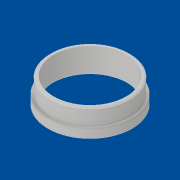
# Autodesk Inventor part: 106-pulley adapter
Saved by Autodesk Inventor 2018 (Build 220112000, 112)
## iProperties
Created: 2020-09-07
Part Number: 106-pulley adapter
Material: Generic
Document SubType Name: Modeling
Designer: Bunny320
Density: 1 g/cm^3
Appearance: Default
Author: Bunny320
Autodesk Inventor part; units mm, degrees
ref_plane "YZ Plane" through (0, 0, 0) normal (1, 0, 0) x (0, 1, 0)
ref_plane "XZ Plane" through (0, 0, 0) normal (0, 1, 0) x (-1, 0, 0)
ref_plane "XY Plane" through (0, 0, 0) normal (0, 0, 1) x (1, 0, 0)
sketch "Sketch1" plane through (0, 0, 0) normal (0, 1, 0) x (-1, 0, 0)
  line L0 (-16, 0) -> (-18.5, 0)
  line L1 (-18.5, 0) -> (-18.5, 4)
  line L2 (-18.5, 4) -> (-17.5, 4)
  line L3 (-17.5, 4) -> (-17.5, 11)
  line L4 (-17.5, 11) -> (-16, 11)
  line L5 (-16, 11) -> (-16, 0)
  line L6 (0, 0) -> (0, 48.5854)
  dimension "d0" = 32
  dimension "d1" = 37
  dimension "d3" = 7
  dimension "d4" = 4
  dimension "d5" = 35
  constraints: 14 end point, 5 perpendicular, 1 horizontal, 1 point on line, 1 vertical
  measures "d0" diameter of L5 L6
  measures "d1" diameter of L1 L6
  measures "d3" distance of L2.end L3.end
  measures "d4" distance of L0.end L1.end
  measures "d5" diameter of L3 L6
revolve "Revolution1" add sketch "Sketch1" angle 360 about axis through (0, 0, 0) along (0, 0, 1)
chamfer "Chamfer1" distance 0.5 angle 45 2 edges at (-16, 0, 0) (-17.5, 0, 11)
body "Solid1"
